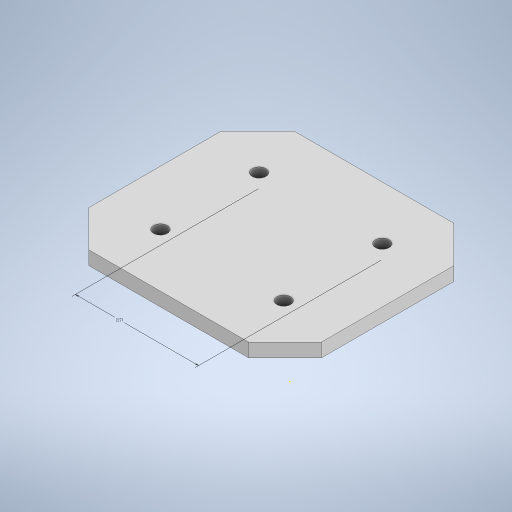
# Autodesk Inventor part: sh2
Saved by Autodesk Inventor 2024 (Build 280153000, 153)
## iProperties
Created: 2023-08-14
Part Number: sh2
Material: 常规
Document SubType Name: Modeling
Designer: wya
Density: 1 g/cm^3
Appearance: 默认
Author: wya
Autodesk Inventor part; units mm, degrees
ref_plane "YZ Plane" through (0, 0, 0) normal (1, 0, 0) x (0, 1, 0)
ref_plane "XZ Plane" through (0, 0, 0) normal (0, 1, 0) x (-1, 0, 0)
ref_plane "XY Plane" through (0, 0, 0) normal (0, 0, 1) x (1, 0, 0)
sketch "草图1" plane through (0, 0, 0) normal (0, 1, 0) x (-1, 0, 0)
  line L0 (0, 0) -> (53, 0)
  line L1 (53, 0) -> (53, -45)
  line L2 (53, -45) -> (0, -45)
  line L3 (0, -45) -> (0, 0)
  line L4 (53, -22.5) -> (49.1677, -22.5)
  line L5 (26.5, -45) -> (26.5, -38.7473)
  circle A0 centre (40, -33.3) radius 1.525
  circle A1 centre (40, -11.7) radius 1.525
  circle A2 centre (13, -33.3) radius 1.525
  circle A3 centre (13, -11.7) radius 1.525
  dimension "d0" = 45
  dimension "d1" = 53
  dimension "d2" = 10.8
  dimension "d3" = 13
  dimension "d4" = 3.05
  constraints: 12 end point, 4 centre point, 2 horizontal, 2 midpoint, 2 parallel, 1 perpendicular, 1 vertical, 3 other
  measures "d0" distance between parallel lines of L2 L0
  measures "d1" distance between parallel lines of L3 L1
  measures "d2" distance from line of L4 A0.centre
  measures "d3" distance from line of L1 A0.centre
  measures "d4" diameter of A0
extrude "拉伸1" add sketch "草图1" along normal blind 3
sketch "草图2" plane through (0, 3, 0) normal (0, 1, 0) x (1, 0, 0)
  line L0 (-52, 50.7806) -> (-1, 50.7806)
  line L1 (-1, 50.7806) -> (-1, -16.6208)
  line L2 (-1, -16.6208) -> (-52, -16.6208)
  line L3 (-52, -16.6208) -> (-52, 50.7806)
  line L4 (-53, 45) -> (-53, 0) projected
  line L5 (0, 0) -> (0, 45) projected
  line L6 (0, 0) -> (0, 45) projected
  line L7 (0, 45) -> (-53, 45) projected
  line L8 (-53, 45) -> (-53, 0) projected
  line L9 (-53, 0) -> (0, 0) projected
  circle A0 centre (-40, 33.3) radius 1.525 projected
  circle A1 centre (-40, 11.7) radius 1.525 projected
  circle A2 centre (-13, 33.3) radius 1.525 projected
  circle A3 centre (-13, 11.7) radius 1.525 projected
  point P0 (-1, 0)
  point P1 (-1, 45)
  point P2 (-52, 0)
  point P3 (-52, 45)
  dimension "d10" = 1
  dimension "d11" = 1
  constraints: 8 end point, 2 parallel, 1 horizontal, 1 perpendicular
  measures "d10" distance between parallel lines of L4 L3
  measures "d11" distance between parallel lines of L5 L1
extrude "拉伸2" cut sketch "草图2" against normal blind 10 contours L3 L9 L4 L7 | L7 L5 L9 L1
chamfer "倒角2" distance 8 angle 45 4 edges at (-1, 1.5, 0) (-52, 1.5, 0) (-52, 1.5, -45) (-1, 1.5, -45)
sketch "草图3" plane through (0, 0, 0) normal (0, -1, 0) x (1, 0, 0)
  circle A0 centre (-40, -33.3) radius 1.525 projected
  circle A1 centre (-13, -33.3) radius 1.525 projected
  point P0 (0, 0)
  dimension "d17" = 27
  measures "d17" distance of A0.centre A1.centre
